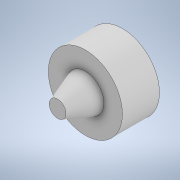
# Autodesk Inventor part: base_product_1
Saved by Autodesk Inventor 2021 (Build 250183000, 183)
## iProperties
Created: 2025-10-28
Part Number: base_product_1
Material: Generic
Document SubType Name: Modeling
Designer: MichaelHanyShawkyHab
Density: 1 g/cm^3
Appearance: Default
Mass: 27.7406 g
Surface Area: 55.0633 cm^2
Volume: 27.7406 cm^3
Author: MichaelHanyShawkyHab
Autodesk Inventor part; units mm, degrees
ref_plane "YZ Plane" through (0, 0, 0) normal (1, 0, 0) x (0, 1, 0)
ref_plane "XZ Plane" through (0, 0, 0) normal (0, 1, 0) x (-1, 0, 0)
ref_plane "XY Plane" through (0, 0, 0) normal (0, 0, 1) x (1, 0, 0)
sketch "Sketch1" plane through (0, 0, 0) normal (0, 0, 1) x (1, 0, 0)
  circle A0 centre (0, 0) radius 20
  dimension "d0" = 40
  constraints: 1 centre point, 1 coincident
  measures "d0" diameter of A0
extrude "Extrusion1" add sketch "Sketch1" along normal blind 20
sketch "Sketch2" plane through (0, 0, 20) normal (0, 0, 1) x (1, 0, 0)
  circle A0 centre (0, 0) radius 10
  dimension "d3" = 20
  constraints: 1 centre point, 1 coincident
  measures "d3" diameter of A0
extrude "Extrusion2" add sketch "Sketch2" along normal blind 15 draft -20
body "Solid1"
